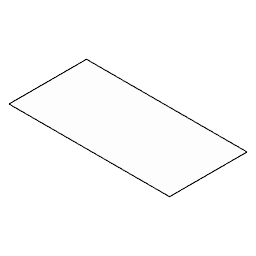
clockAssembly (Autodesk Fusion 360 archive; units mm, degrees)
design "glass sheet"
part number: 2026-06-02-13-22-38-638
Autodesk Fusion 360 part; units mm, degrees
sketch "Sketch1" plane through (0, 0, 0) normal (0, 0, 1) x (1, 0, 0)
  line L0 (-36.2469, 42.7798) -> (253.7531, 42.7798)
  line L1 (253.7531, 42.7798) -> (253.7531, -97.2202)
  line L2 (253.7531, -97.2202) -> (-36.2469, -97.2202)
  line L3 (-36.2469, -97.2202) -> (-36.2469, 42.7798)
  dimension "d1" = 290
  dimension "d2" = 140
  constraint horizontal L0
  constraint vertical L1
  constraint horizontal L2
  constraint vertical L3
  measures "d1" distance of L0.start L0.end
  measures "d2" distance of L0.start L2.end
extrude "Extrude1" add sketch "Sketch1" along normal blind 0.2

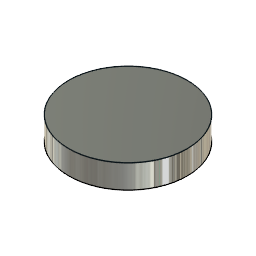
design "neodymium magnets 5x1"
part number: 2026-05-31-08-33-18-494
Autodesk Fusion 360 part; units mm, degrees
sketch "Sketch1" plane through (0, 0, 0) normal (0, 0, 1) x (1, 0, 0)
  circle A0 centre (0, 0) radius 2.5
  dimension "d1" = 5
  constraint coincident A0.centre origin
  measures "d1" diameter of A0
extrude "Extrude1" add sketch "Sketch1" along normal blind 1
sketch "Sketch2" plane through (0, 0, 1) normal (0, 0, 1) x (-1, 0, 0)
  circle A0 centre (0, 0) radius 2.5
sketch "Sketch3" plane through (0, 0, 0) normal (0, 1, 0) x (1, 0, 0)
